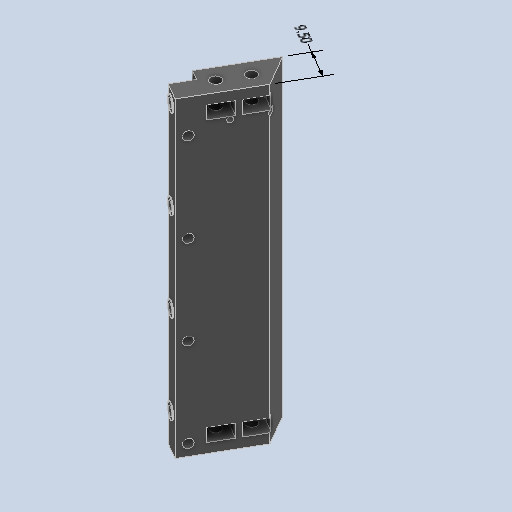
# Autodesk Inventor part: base_bearingpole_side
Saved by Autodesk Inventor 2024.1 (Build 281209000, 209)
## iProperties
Created: 2025-01-17
Part Number: base_bearingpole_side
Material: 一般
Document SubType Name: Modeling
Designer: hibik
Density: 1 g/cm^3
Appearance: 既定
Author: hibik
Autodesk Inventor part; units mm, degrees
ref_plane "YZ Plane" through (0, 0, 0) normal (1, 0, 0) x (0, 1, 0)
ref_plane "XZ Plane" through (0, 0, 0) normal (0, 1, 0) x (-1, 0, 0)
ref_plane "XY Plane" through (0, 0, 0) normal (0, 0, 1) x (1, 0, 0)
sketch "スケッチ1" plane through (0, 0, 0) normal (0, 1, 0) x (-1, 0, 0)
  line L0 (8.2272, -4.75) -> (0, 0)
  line L1 (0, 0) -> (-10.8031, -18.7115)
  line L2 (-10.8031, -18.7115) -> (-5.3183, -28.2115)
  line L3 (-5.3183, -28.2115) -> (8.2272, -4.75)
  line L4 (31.5369, 0) -> (-17.8598, 0) projected
  line L5 (0, 0) -> (19.1969, 33.25)
  line L6 (19.1969, 33.25) -> (24.4803, 30.1996) construction
  line L7 (5.1962, -3) -> (1.9462, -8.6292)
  line L8 (1.9462, -8.6292) -> (4.9772, -10.3792)
  dimension "d0" = 9.5
  dimension "d2" = 60
  dimension "d3" = 60
  dimension "d4" = 60
  dimension "d8" = 38
  dimension "d9" = 3.5
  dimension "d10" = 6.5
  constraints: 16 end point, 5 perpendicular, 2 point on line, 1 collinear
  measures "d0" distance of L0.end L0.start
  measures "d2" angle of L4 L1
  measures "d3" angle of L4 L2
  measures "d4" distance from line of L1.end L6
  measures "d8" vertical distance of L0.start L5.end
  measures "d9" distance between parallel lines of L3 L7
  measures "d10" distance from line of L7.start L8
extrude "押し出し1" add sketch "スケッチ1" along normal blind 97 contours L7 L8 L3 L2 L1 L0
sketch "スケッチ2" plane through (-5.1962, 0, -3) normal (-0.8660254, 0, -0.5) x (-0.5, 0, 0.8660254)
  circle A0 centre (-3, 3.5) radius 3
  line L0 (-6.5, 0) -> (0, 0) projected
  line L1 (0, 0) -> (0, 97) projected
  circle A1 centre (-3, 3.5) radius 1.35
  dimension "d12" = 6
  dimension "d13" = 3.5
  dimension "d14" = 2.7
  constraints: 2 centre point, 1 coincident, 1 tangent
  measures "d12" diameter of A0
  measures "d13" distance from line of L0 A0.centre
  measures "d14" diameter of A1
extrude "押し出し2" cut sketch "スケッチ2" against normal through all contours A1
sketch "スケッチ3" plane through (-5.1962, 0, -3) normal (-0.8660254, 0, -0.5) x (-0.5, 0, 0.8660254)
  circle A0 centre (-3, 3.5) radius 1.35 projected
  circle A1 centre (-3, 3.5) radius 2.25
  point P0 (0, 0)
  dimension "d17" = 4.5
  constraints: 1 centre point, 1 coincident
  measures "d17" diameter of A1
extrude "押し出し3" add sketch "スケッチ3" along normal blind 0.5
sketch "スケッチ4" plane through (0, 0, 0) normal (-0.5, 0, 0.8660254) x (0.8660254, 0, 0.5)
  circle A0 centre (-3.5, 10.5) radius 3
  line L0 (-6, 0) -> (-6, 97) projected
  line L1 (-6, 7) -> (0, 7)
  line L2 (-6, 0) -> (0, 0) projected
  line L3 (-9.5, 0) -> (-6, 0) projected
  line L4 (-6.5, 0) -> (-6.5, 11.2829)
  circle A1 centre (-3.5, 10.5) radius 1.35
  dimension "d20" = 6
  dimension "d21" = 7
  dimension "d22" = 3.5
  dimension "d23" = 0.5
  dimension "d24" = 2.7
  constraints: 4 end point, 2 centre point, 2 point on line, 1 coincident, 1 horizontal, 1 perpendicular, 1 tangent
  measures "d20" diameter of A0
  measures "d21" distance between parallel lines of L2 L1
  measures "d22" distance from line of A0.centre L1
  measures "d23" distance between parallel lines of L0 L4
  measures "d24" diameter of A1
extrude "押し出し4" cut sketch "スケッチ4" against normal blind 5 contours A1
sketch "スケッチ5" plane through (0, 0, 0) normal (-0.5, 0, 0.8660254) x (0.8660254, 0, 0.5)
  circle A0 centre (-3.5, 10.5) radius 1.35 projected
  circle A1 centre (-3.5, 10.5) radius 2.25
  point P0 (0, 0)
  dimension "d27" = 4.5
  constraints: 1 centre point, 1 coincident
  measures "d27" diameter of A1
extrude "押し出し5" add sketch "スケッチ5" along normal blind 0.2
pattern_linear "矩形状パターン1" count 4 spacing 27.6667 along (0, 1, 0) of "押し出し2", "押し出し3", "押し出し4", "押し出し5"
sketch "スケッチ6" plane through (-4.9772, 0, -10.3792) normal (-0.8660254, 0, -0.5) x (-0.5, 0, 0.8660254)
  line L0 (-20.591, 0) -> (-20.591, 97) projected
  line L1 (-20.591, 96) -> (-1.091, 96)
  line L2 (-1.091, 96) -> (-1.091, 81.4)
  line L3 (-1.091, 81.4) -> (-20.591, 81.4)
  line L4 (-20.591, 81.4) -> (-20.591, 96)
  line L5 (-20.591, 97) -> (0, 97) projected
  line L6 (-20.591, 96) -> (-1.091, 96)
  line L7 (-1.091, 96) -> (-1.091, 97)
  line L8 (-1.091, 97) -> (-20.591, 97)
  line L9 (-20.591, 97) -> (-20.591, 96)
  circle A0 centre (-15.591, 89.1) radius 0.85
  circle A1 centre (-6.091, 89.1) radius 0.85
  line L10 (-10.841, 81.4) -> (-10.841, 96)
  point P0 (6.5, 0)
  point P1 (-1.091, 96)
  dimension "d33" = 19.5
  dimension "d34" = 14.6
  dimension "d35" = 1
  dimension "d36" = 1.7
  dimension "d37" = 6.9
  dimension "d38" = 9.5
  constraints: 18 end point, 4 parallel, 2 centre point, 2 horizontal, 2 midpoint, 2 perpendicular, 2 point on line, 1 collinear, 1 equal radius, 1 symmetric about line
  measures "d33" distance of L2.end L3.end
  measures "d34" distance between parallel lines of L3 L1
  measures "d35" distance between parallel lines of L5 L1
  measures "d36" diameter of A0
  measures "d37" distance from line of L1 A0.centre
  measures "d38" distance of A1.centre A0.centre
extrude "押し出し6" cut sketch "スケッチ6" against normal through all contours A0 | A1
sketch "スケッチ8" plane through (0, 97, 0) normal (0, 1, 0) x (1, 0, 0)
  line L0 (4.5139, 11.4183) -> (2.8684, 8.5683)
  line L1 (2.8684, 8.5683) -> (-0.4225, 8.5683)
  line L2 (-0.4225, 8.5683) -> (-2.0679, 11.4183)
  line L3 (-2.0679, 11.4183) -> (-0.4225, 14.2683)
  line L4 (-0.4225, 14.2683) -> (2.8684, 14.2683)
  line L5 (2.8684, 14.2683) -> (4.5139, 11.4183)
  line L6 (6.9637, 15.6615) -> (3.6728, 15.6615)
  line L7 (3.6728, 15.6615) -> (2.0274, 18.5115)
  line L8 (2.0274, 18.5115) -> (3.6728, 21.3615)
  line L9 (3.6728, 21.3615) -> (6.9637, 21.3615)
  line L10 (6.9637, 21.3615) -> (8.6092, 18.5115)
  line L11 (8.6092, 18.5115) -> (6.9637, 15.6615)
  line L12 (5.3183, 28.2115) -> (-4.9772, 10.3792) projected
  line L13 (10.8031, 18.7115) -> (5.3183, 28.2115) projected
  line L14 (-4.9772, 10.3792) -> (-1.9462, 8.6292) projected
  line L15 (-0.4225, 8.5683) -> (3.6046, 6.2433)
  line L16 (0, 0) -> (10.8031, 18.7115) projected
  line L17 (2.8684, 14.2683) -> (6.8954, 11.9433)
  line L18 (3.6728, 15.6615) -> (7.6998, 13.3365)
  line L19 (6.9637, 21.3615) -> (11.0441, 19.0057)
  circle A0 centre (1.223, 11.4183) radius 1.6
  circle A1 centre (5.3183, 18.5115) radius 1.6
  point P0 (10.4278, 19.3615)
  dimension "d47" = 5.7
  dimension "d48" = 2
  dimension "d49" = 2
  dimension "d50" = 4
  dimension "d51" = 3.2
  dimension "d52" = 3.2
  constraints: 32 end point, 3 perpendicular, 3 point on line, 2 centre point, 2 coincident, 2 collinear, 2 parallel, 26 other
  measures "d47" distance between parallel lines of L11 L8
  measures "d48" distance between parallel lines of L12 L8
  measures "d49" distance between parallel lines of L13 L10
  measures "d50" distance from line of L14 point (1.223, 11.418)
  measures "d51" diameter of A0
  measures "d52" diameter of A1
extrude "押し出し8" cut sketch "スケッチ8" against normal blind 15 contours A0 | A1
extrude "押し出し9" cut sketch "スケッチ8" against normal blind 7
extrude "押し出し10" add sketch "スケッチ8" against normal blind 3
ref_plane "作業平面1" through (0, 48.5, 0) normal (0, 1, 0) x (1, 0, 0)
mirror "ミラー1" about plane through (0, 48.5, 0) normal (0, 1, 0) of "押し出し8", "押し出し9", "押し出し10"
